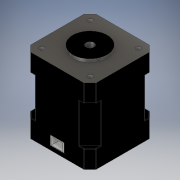
# Autodesk Inventor part: Stepper Motor
Saved by Autodesk Inventor 2018 (Build 220112000, 112)
## iProperties
Created: 2018-03-28
Part Number: Stepper Motor
Material: Generic
Document SubType Name: Modeling
Designer: Ajith Thomas
Density: 1 g/cm^3
Appearance: Default
Author: Ajith Thomas
Autodesk Inventor part; units mm, degrees
ref_plane "YZ Plane" through (0, 0, 0) normal (1, 0, 0) x (0, 1, 0)
ref_plane "XZ Plane" through (0, 0, 0) normal (0, 1, 0) x (-1, 0, 0)
sketch "Sketch1" plane through (0, 0, 0) normal (0, 1, 0) x (-1, 0, 0)
  line L0 (17, 21) -> (-17, 21)
  line L1 (-21, 17) -> (-21, -17)
  line L2 (-17, -21) -> (17, -21)
  line L3 (21, -17) -> (21, 17)
  line L4 (21, 21) -> (-21, -21) construction
  line L5 (-21, 21) -> (21, -21) construction
  line L6 (21, 0) -> (-21, 0) construction
  line L7 (0, 21) -> (0, -21) construction
  line L8 (0, -21) -> (17, -21) construction
  line L9 (21, 0) -> (21, -17) construction
  line L10 (21, -17) -> (17, -21)
  line L11 (21, 17) -> (17, 21)
  line L12 (-21, -17) -> (-17, -21)
  line L13 (-21, 17) -> (-17, 21)
  point P0 (0, 0)
  dimension "d0" = 42
  dimension "d1" = 42
  dimension "d2" = 17
  dimension "d3" = 17
  constraints: 28 end point, 6 midpoint, 6 symmetric about line, 2 parallel, 1 horizontal, 1 perpendicular
  measures "d0" distance of L5.end L4.end
  measures "d1" distance of L4.end L5.start
  measures "d2" distance of L2.end L7.end
  measures "d3" distance of L3.start L6.start
extrude "Extrusion1" add sketch "Sketch1" along normal blind 48
ref_plane "Work Plane1" through (0, 24, 0) normal (0, 1, 0) x (1, 0, 0)
sketch "Sketch2" plane through (0, 24, 0) normal (0, 1, 0) x (1, 0, 0)
  line L0 (17, -21) -> (-17, -21) projected
  line L1 (-17, -21) -> (-21, -17) projected
  line L2 (-21, -17) -> (-21, 17) projected
  line L3 (-21, 17) -> (-17, 21) projected
  line L4 (-17, 21) -> (17, 21) projected
  line L5 (17, 21) -> (21, 17) projected
  line L6 (21, 17) -> (21, -17) projected
  line L7 (21, -17) -> (17, -21) projected
  line L8 (0, 21) -> (0, -21) construction
  line L9 (17, -21) -> (-17, -21) construction
  line L10 (-21, -17) -> (-21, 17) construction
  line L11 (-21, 0) -> (21, 0) construction
  line L12 (0, 21) -> (14, 21) construction
  line L13 (-17, 21) -> (17, 21) construction
  line L14 (21, 0) -> (21, 14) construction
  line L15 (21, 17) -> (21, -17) construction
  line L16 (14, 21) -> (21, 14)
  line L17 (-14, 21) -> (-21, 14)
  line L18 (14, -21) -> (21, -14)
  line L19 (-14, -21) -> (-21, -14)
  line L20 (14, -21) -> (17, -21)
  line L21 (21, -17) -> (17, -21) projected
  line L22 (21, -17) -> (21, -14)
  line L23 (17, -21) -> (21, -17)
  line L24 (17, 21) -> (21, 17) projected
  line L25 (21, 14) -> (21, 17)
  line L26 (21, 17) -> (17, 21)
  line L27 (17, 21) -> (14, 21)
  line L28 (-14, 21) -> (-17, 21)
  line L29 (-21, 17) -> (-17, 21) projected
  line L30 (-21, 17) -> (-21, 14)
  line L31 (-17, 21) -> (-21, 17)
  line L32 (-14, -21) -> (-17, -21)
  line L33 (-17, -21) -> (-21, -17) projected
  line L34 (-21, -17) -> (-21, -14)
  line L35 (-17, -21) -> (-21, -17)
  point P0 (0, 0)
  dimension "d6" = 14
  dimension "d7" = 14
  constraints: 40 end point, 7 collinear, 6 symmetric about line, 4 midpoint, 4 perpendicular, 2 point on line, 1 vertical
  measures "d6" distance of L8.start L12.end
  measures "d7" distance of L11.end L14.end
extrude "Extrusion2" cut sketch "Sketch2" along normal mid plane 25 contours L0 L18 L6 L7 | L0 L1 L2 L19 | L16 L4 L5 L6 | L2 L3 L4 L17
sketch "Sketch3" plane through (0, 48, 0) normal (0, 1, 0) x (1, 0, 0)
  circle A0 centre (0, 0) radius 11
  dimension "d10" = 22
  constraints: 1 centre point, 1 coincident
  measures "d10" diameter of A0
extrude "Extrusion3" add sketch "Sketch3" along normal blind 2
sketch "Sketch4" plane through (0, 50, 0) normal (0, 1, 0) x (1, 0, 0)
  circle A0 centre (0, 0) radius 2.5
  dimension "d13" = 5
  constraints: 1 centre point, 1 coincident
  measures "d13" diameter of A0
extrude "Extrusion4" cut sketch "Sketch4" against normal blind 70.2625
sketch "Sketch5" plane through (0, 48, 0) normal (0, 1, 0) x (1, 0, 0)
  line L0 (21, -17) -> (21, 17) construction
  line L1 (-17, -21) -> (17, -21) construction
  line L2 (17, 21) -> (-17, 21) construction
  line L3 (-21, 17) -> (-21, -17) construction
  line L4 (0, 21) -> (0, -21) construction
  line L5 (17, -21) -> (-17, -21) construction
  line L6 (21, 0) -> (-21, 0) construction
  line L7 (-21, -17) -> (-21, 17) construction
  circle A0 centre (15.5, -15.5) radius 1.5
  circle A1 centre (15.5, 15.5) radius 1.5
  circle A2 centre (-15.5, -15.5) radius 1.5
  circle A3 centre (-15.5, 15.5) radius 1.5
  point P0 (0, 0)
  dimension "d16" = 3
  dimension "d17" = 15.5
  dimension "d18" = 15.5
  constraints: 4 centre point, 4 end point, 4 midpoint, 3 symmetric about line, 3 other
  measures "d16" diameter of A0
  measures "d17" horizontal distance of A0.centre point (0, 0)
  measures "d18" horizontal distance of A0.centre point (0, 0)
extrude "Extrusion5" cut sketch "Sketch5" against normal blind 4.5
thread "Thread1" size "M3x0.5" class "6H" standard "ANSI Metric M Profile" full length
thread "Thread2" size "M3x0.5" class "6H" standard "ANSI Metric M Profile" full length
thread "Thread3" size "M3x0.5" class "6H" standard "ANSI Metric M Profile" full length
thread "Thread4" size "M3x0.5" class "6H" standard "ANSI Metric M Profile" full length
sketch "Sketch6" plane through (0, 0, 0) normal (0, -1, 0) x (1, 0, 0)
  circle A0 centre (15.5, -15.5) radius 1.5 projected
  circle A1 centre (15.5, 15.5) radius 1.5 projected
  circle A2 centre (-15.5, 15.5) radius 1.5 projected
  circle A3 centre (-15.5, -15.5) radius 1.5 projected
  point P0 (0, 0)
extrude "Extrusion6" cut sketch "Sketch6" against normal blind 10
sketch "Sketch7" plane through (0, 0, 0) normal (0, -1, 0) x (1, 0, 0)
  circle A0 centre (15.5, 15.5) radius 1.5 projected
  circle A1 centre (15.5, 15.5) radius 3
  circle A2 centre (15.5, -15.5) radius 1.5 projected
  circle A3 centre (15.5, -15.5) radius 3
  circle A4 centre (-15.5, -15.5) radius 1.5 projected
  circle A5 centre (-15.5, -15.5) radius 3
  circle A6 centre (-15.5, 15.5) radius 1.5 projected
  circle A7 centre (-15.5, 15.5) radius 3
  point P0 (0, 0)
  dimension "d31" = 6
  dimension "d32" = 6
  dimension "d33" = 6
  dimension "d35" = 6
  constraints: 4 centre point, 4 coincident
  measures "d31" diameter of A1
  measures "d32" diameter of A3
  measures "d33" diameter of A5
  measures "d35" diameter of A7
extrude "Extrusion7" cut sketch "Sketch7" against normal blind 2
fillet "Fillet1" radius 0.3 48 edges at (-21, 42.25, -17) (-17, 42.25, -21) (-19, 36.5, -19) (-21, 24, -14) (-14, 24, -21) (-19, 11.5, -19) (-17, 5.75, -21) (-21, 5.75, -17) (-21, 11.5, -15.5) (-15.5, 11.5, -21) (-21, 36.5, -15.5) (-15.5, 36.5, -21) (-17, 5.75, 21) (-21, 5.75, 17) (-19, 11.5, 19) (-21, 11.5, 15.5) (-15.5, 11.5, 21) (-14, 24, 21) (-21, 24, 14) (-19, 36.5, 19) (-21, 42.25, 17) (-17, 42.25, 21) (-21, 36.5, 15.5) (-15.5, 36.5, 21) (17, 42.25, 21) (21, 42.25, 17) (21, 36.5, 15.5) (19, 36.5, 19) (15.5, 36.5, 21) (14, 24, 21) (21, 24, 14) (21, 11.5, 15.5) (19, 11.5, 19) (15.5, 11.5, 21) (17, 5.75, 21) (21, 5.75, 17) (21, 42.25, -17) (17, 42.25, -21) (21, 24, -14) (14, 24, -21) (21, 5.75, -17) (17, 5.75, -21) (15.5, 11.5, -21) (19, 11.5, -19) (21, 11.5, -15.5) (21, 36.5, -15.5) (19, 36.5, -19) (15.5, 36.5, -21)
sketch "Sketch8" plane through (-16.8757, 0, 21) normal (0, 0, 1) x (1, 0, 0)
  line L0 (33.7515, 0) -> (0, 0) projected
  line L1 (0, 48) -> (33.7515, 48) projected
  line L2 (5.8757, 48) -> (27.8757, 48) construction
  line L3 (16.8757, 48) -> (16.8757, 0) construction
  line L4 (12.3757, 8.5) -> (21.3757, 8.5)
  line L5 (21.3757, 8.5) -> (21.3757, 2.5)
  line L6 (21.3757, 2.5) -> (12.3757, 2.5)
  line L7 (12.3757, 2.5) -> (12.3757, 8.5)
  line L8 (12.3757, 8.5) -> (21.3757, 2.5) construction
  line L9 (21.3757, 8.5) -> (12.3757, 2.5) construction
  point P0 (16.8757, 5.5)
  dimension "d39" = 9
  dimension "d40" = 6
  dimension "d41" = 2.5
  constraints: 14 end point, 3 midpoint, 2 parallel, 2 perpendicular, 1 horizontal, 1 point on line
  measures "d39" distance of L5.end L6.end
  measures "d40" distance of L4.end L5.end
  measures "d41" distance between parallel lines of L0 L6
extrude "Extrusion8" cut sketch "Sketch8" against normal blind 5
sketch "Sketch9" plane through (-16.8757, 0, 16) normal (0, 0, 1) x (1, 0, 0)
  line L0 (12.3757, 8.5) -> (21.3757, 8.5) projected
  line L1 (21.3757, 8.5) -> (21.3757, 2.5) projected
  line L2 (21.3757, 2.5) -> (12.3757, 2.5) projected
  line L3 (12.3757, 2.5) -> (12.3757, 8.5) projected
  line L4 (12.3757, 8.5) -> (21.3757, 8.5) construction
  line L5 (16.8757, 8.5) -> (16.8757, 2.5) construction
  line L6 (21.3757, 2.5) -> (12.3757, 2.5) construction
  line L7 (12.3757, 2.5) -> (12.3757, 8.5) construction
  line L8 (12.3757, 5.5) -> (21.3757, 5.5) construction
  line L9 (12.6206, 8.2381) -> (21.1309, 8.2381)
  line L10 (21.1309, 8.2381) -> (21.1309, 2.7619)
  line L11 (21.1309, 2.7619) -> (12.6206, 2.7619)
  line L12 (12.6206, 2.7619) -> (12.6206, 8.2381)
  line L13 (12.6206, 8.2381) -> (21.1309, 2.7619) construction
  line L14 (21.1309, 8.2381) -> (12.6206, 2.7619) construction
  line L15 (13.2708, 7.8197) -> (20.4807, 7.8197)
  line L16 (20.4807, 7.8197) -> (20.4807, 3.1803)
  line L17 (20.4807, 3.1803) -> (13.2708, 3.1803)
  line L18 (13.2708, 3.1803) -> (13.2708, 7.8197)
  line L19 (13.2708, 7.8197) -> (20.4807, 3.1803) construction
  line L20 (20.4807, 7.8197) -> (13.2708, 3.1803) construction
  point P0 (16.8757, 0)
  point P1 (16.8757, 5.5)
  point P2 (16.8757, 5.5)
  constraints: 28 end point, 10 midpoint, 4 parallel, 2 horizontal, 2 perpendicular, 1 point on line
extrude "Extrusion9" add sketch "Sketch9" along normal blind 5 contours L9 L10 L11 L12
body "Solid1"
